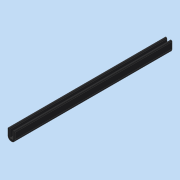
# Autodesk Inventor part: 0 零件
Saved by Autodesk Inventor 2020 (Build 240168000, 168)
## iProperties
Created: 2020-11-03
Part Number: 0 零件
Material: 橡膠
Document SubType Name: Modeling
Designer: p2013
Density: 0.93 g/cm^3
Appearance: 橡膠 - 黑色
Author: p2013
Autodesk Inventor part; units mm, degrees
ref_plane "YZ Plane" through (0, 0, 0) normal (1, 0, 0) x (0, 1, 0)
ref_plane "XZ Plane" through (0, 0, 0) normal (0, 1, 0) x (-1, 0, 0)
ref_plane "XY Plane" through (0, 0, 0) normal (0, 0, 1) x (1, 0, 0)
sketch "草圖1" plane through (0, 0, 0) normal (0, 0, 1) x (1, 0, 0)
  line L0 (0, 0) -> (-19.4073, 0) construction
  line L1 (0, 0) -> (0, 21.4127) construction
  line L2 (-3, 8.125) -> (-3, 3)
  arc A0 (-3, 3) -> (3, 3) centre (0, 3) ccw
  line L3 (3, 3) -> (3, 8.125)
  line L4 (1.25, 8.125) -> (1.25, 2)
  line L5 (-1.25, 2) -> (-1.25, 8.125)
  line L6 (-3, 9.712) -> (-3, 6.8385) construction
  line L7 (3, 9.712) -> (3, 6.8385) construction
  line L8 (-4.0339, 9) -> (4.2037, 9) construction
  line L9 (-1.25, 2) -> (1.25, 2)
  arc A1 (-1.25, 8.125) -> (-3, 8.125) centre (-2.125, 8.125) ccw
  arc A2 (3, 8.125) -> (1.25, 8.125) centre (2.125, 8.125) ccw
  dimension "d0" = 6
  dimension "d2" = 9
  dimension "d3" = 2
  dimension "d4" = 2.5
  dimension "d6" = 6
  constraints: 20 end point, 6 point on circle, 6 tangent, 5 symmetric about line, 3 centre point, 3 horizontal, 3 vertical, 1 point on line, 3 other
  measures "d0" distance between parallel lines of L7 L6
  measures "d2" distance between parallel lines of L0 L8
  measures "d3" distance from line of L0.start L9
  measures "d4" distance of L5.start L4.end
  measures "d6" distance of L3.start L2.end
extrude "擠出1" add sketch "草圖1" along normal mid plane 130
